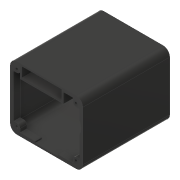
# Autodesk Inventor part: Case for Fan
Saved by Autodesk Inventor 2017 (Build 210142000, 142)
## iProperties
Created: 2016-08-11
Part Number: Case for Fan
Material: Generic
Document SubType Name: Modeling
Designer: ge937963
Density: 1 g/cm^3
Appearance: Smooth - Black
Mass: 36.4962 g
Surface Area: 460.668 cm^2
Volume: 36.4962 cm^3
Author: ge937963
Autodesk Inventor part; units mm, degrees
(part 1 of 2)
sketch "Sketch1" plane through (0, 0, 0) normal (0, 0, 1) x (1, 0, 0)
  line L0 (-32.8456, -23.6218) -> (-32.8456, 23.6218) projected
  arc A0 (-28.0831, 28.3843) -> (-32.8456, 23.6218) centre (-28.0831, 23.6218) ccw projected
  line L1 (-28.0831, 28.3843) -> (28.0831, 28.3843) projected
  arc A1 (32.8456, 23.6218) -> (28.0831, 28.3843) centre (28.0831, 23.6218) ccw projected
  line L2 (32.8456, 23.6218) -> (32.8456, -23.6218) projected
  arc A2 (28.0831, -28.3843) -> (32.8456, -23.6218) centre (28.0831, -23.6218) ccw projected
  line L3 (28.0831, -28.3843) -> (-28.0831, -28.3843) projected
  arc A3 (-32.8456, -23.6218) -> (-28.0831, -28.3843) centre (-28.0831, -23.6218) ccw projected
  arc A4 (-34.4331, -23.6218) -> (-28.0831, -29.9718) centre (-28.0831, -23.6218) ccw projected
  line L4 (-28.0831, -29.9718) -> (28.0831, -29.9718) projected
  arc A5 (28.0831, -29.9718) -> (34.4331, -23.6218) centre (28.0831, -23.6218) ccw projected
  line L5 (34.4331, -23.6218) -> (34.4331, 23.6218) projected
  arc A6 (34.4331, 23.6218) -> (28.0831, 29.9718) centre (28.0831, 23.6218) ccw projected
  line L6 (28.0831, 29.9718) -> (-28.0831, 29.9718) projected
  arc A7 (-28.0831, 29.9718) -> (-34.4331, 23.6218) centre (-28.0831, 23.6218) ccw projected
  line L7 (-34.4331, 23.6218) -> (-34.4331, -23.6218) projected
  point P0 (0, 0)
extrude "Extrusion1" add sketch "Sketch1" along normal blind 82.55
sketch "Sketch2" plane through (0, 0, 0) normal (0, 0, -1) x (-1, 0, 0)
  line L0 (32.8456, -23.6218) -> (32.8456, 23.6218) projected
  arc A0 (32.8456, 23.6218) -> (28.0831, 28.3843) centre (28.0831, 23.6218) ccw projected
  line L1 (28.0831, 28.3843) -> (-28.0831, 28.3843) projected
  arc A1 (-28.0831, 28.3843) -> (-32.8456, 23.6218) centre (-28.0831, 23.6218) ccw projected
  line L2 (-32.8456, 23.6218) -> (-32.8456, -23.6218) projected
  arc A2 (-32.8456, -23.6218) -> (-28.0831, -28.3843) centre (-28.0831, -23.6218) ccw projected
  line L3 (-28.0831, -28.3843) -> (28.0831, -28.3843) projected
  arc A3 (28.0831, -28.3843) -> (32.8456, -23.6218) centre (28.0831, -23.6218) ccw projected
  arc A4 (28.0831, -29.9718) -> (34.4331, -23.6218) centre (28.0831, -23.6218) ccw projected
  line L4 (28.0831, -29.9718) -> (-28.0831, -29.9718) projected
  arc A5 (-34.4331, -23.6218) -> (-28.0831, -29.9718) centre (-28.0831, -23.6218) ccw projected
  line L5 (-34.4331, -23.6218) -> (-34.4331, 23.6218) projected
  arc A6 (-28.0831, 29.9718) -> (-34.4331, 23.6218) centre (-28.0831, 23.6218) ccw projected
  line L6 (-28.0831, 29.9718) -> (28.0831, 29.9718) projected
  arc A7 (34.4331, 23.6218) -> (28.0831, 29.9718) centre (28.0831, 23.6218) ccw projected
  line L7 (34.4331, 23.6218) -> (34.4331, -23.6218) projected
  arc A8 (28.0831, -26.5428) -> (31.0041, -23.6218) centre (28.0831, -23.6218) ccw projected
  arc A9 (-31.0041, -23.6218) -> (-28.0831, -26.5428) centre (-28.0831, -23.6218) ccw projected
  arc A10 (-28.0831, 26.5428) -> (-31.0041, 23.6218) centre (-28.0831, 23.6218) ccw projected
  arc A11 (31.0041, 23.6218) -> (28.0831, 26.5428) centre (28.0831, 23.6218) ccw projected
  line L8 (32.4646, -23.6218) -> (32.4646, 23.6218)
  arc A12 (32.4646, 23.6218) -> (28.0831, 28.0033) centre (28.0831, 23.6218) ccw
  line L9 (28.0831, 28.0033) -> (-28.0831, 28.0033)
  arc A13 (-28.0831, 28.0033) -> (-32.4646, 23.6218) centre (-28.0831, 23.6218) ccw
  line L10 (-32.4646, 23.6218) -> (-32.4646, -23.6218)
  arc A14 (-32.4646, -23.6218) -> (-28.0831, -28.0033) centre (-28.0831, -23.6218) ccw
  line L11 (-28.0831, -28.0033) -> (28.0831, -28.0033)
  arc A15 (28.0831, -28.0033) -> (32.4646, -23.6218) centre (28.0831, -23.6218) ccw
  line L12 (28.0831, -26.5428) -> (-28.0831, -26.5428)
  line L13 (-31.0041, -23.6218) -> (-31.0041, 23.6218)
  line L14 (-28.0831, 26.5428) -> (28.0831, 26.5428)
  line L15 (31.0041, 23.6218) -> (31.0041, -23.6218)
  arc A16 (-31.3851, -23.6218) -> (-28.0831, -26.9238) centre (-28.0831, -23.6218) ccw
  line L16 (-31.3851, -23.6218) -> (-31.3851, 23.6218)
  arc A17 (-28.0831, 26.9238) -> (-31.3851, 23.6218) centre (-28.0831, 23.6218) ccw
  line L17 (-28.0831, 26.9238) -> (28.0831, 26.9238)
  arc A18 (31.3851, 23.6218) -> (28.0831, 26.9238) centre (28.0831, 23.6218) ccw
  line L18 (31.3851, 23.6218) -> (31.3851, -23.6218)
  arc A19 (28.0831, -26.9238) -> (31.3851, -23.6218) centre (28.0831, -23.6218) ccw
  line L19 (28.0831, -26.9238) -> (-28.0831, -26.9238)
  point P0 (0, 0)
  dimension "d2" = 0.381
  dimension "d3" = 0.381
  constraints: 24 end point, 16 point on circle, 8 centre point, 4 perpendicular, 2 tangent, 1 horizontal, 1 parallel, 14 other
  measures "d2" distance between parallel lines of L3 L11
  measures "d3" distance between parallel lines of L12 L19
extrude "Extrusion2" add sketch "Sketch2" along normal blind 3.175 contours A15 L11 A14 L10 A13 L9 A12 L8
sketch "Sketch3" plane through (0, 0, 0) normal (0, 0, 1) x (1, 0, 0)
  line L0 (31.3851, 23.6218) -> (31.3851, -23.6218) projected
  arc A0 (28.0831, -26.9238) -> (31.3851, -23.6218) centre (28.0831, -23.6218) ccw projected
  line L1 (28.0831, -26.9238) -> (-28.0831, -26.9238) projected
  arc A1 (-31.3851, -23.6218) -> (-28.0831, -26.9238) centre (-28.0831, -23.6218) ccw projected
  line L2 (-31.3851, -23.6218) -> (-31.3851, 23.6218) projected
  arc A2 (-28.0831, 26.9238) -> (-31.3851, 23.6218) centre (-28.0831, 23.6218) ccw projected
  line L3 (-28.0831, 26.9238) -> (28.0831, 26.9238) projected
  arc A3 (31.3851, 23.6218) -> (28.0831, 26.9238) centre (28.0831, 23.6218) ccw projected
  line L4 (-32.4646, -23.6218) -> (-32.4646, 23.6218) projected
  arc A4 (-32.4646, -23.6218) -> (-28.0831, -28.0033) centre (-28.0831, -23.6218) ccw projected
  line L5 (28.0831, -28.0033) -> (-28.0831, -28.0033) projected
  arc A5 (28.0831, -28.0033) -> (32.4646, -23.6218) centre (28.0831, -23.6218) ccw projected
  line L6 (32.4646, 23.6218) -> (32.4646, -23.6218) projected
  arc A6 (32.4646, 23.6218) -> (28.0831, 28.0033) centre (28.0831, 23.6218) ccw projected
  line L7 (-28.0831, 28.0033) -> (28.0831, 28.0033) projected
  arc A7 (-28.0831, 28.0033) -> (-32.4646, 23.6218) centre (-28.0831, 23.6218) ccw projected
  arc A8 (-28.0831, 28.3843) -> (-32.8456, 23.6218) centre (-28.0831, 23.6218) ccw projected
  line L8 (-28.0831, 28.3843) -> (28.0831, 28.3843) projected
  arc A9 (32.8456, 23.6218) -> (28.0831, 28.3843) centre (28.0831, 23.6218) ccw projected
  line L9 (32.8456, 23.6218) -> (32.8456, -23.6218) projected
  arc A10 (28.0831, -28.3843) -> (32.8456, -23.6218) centre (28.0831, -23.6218) ccw projected
  line L10 (28.0831, -28.3843) -> (-28.0831, -28.3843) projected
  arc A11 (-32.8456, -23.6218) -> (-28.0831, -28.3843) centre (-28.0831, -23.6218) ccw projected
  line L11 (-32.8456, -23.6218) -> (-32.8456, 23.6218) projected
  arc A12 (-34.4331, -23.6218) -> (-28.0831, -29.9718) centre (-28.0831, -23.6218) ccw projected
  line L12 (-28.0831, -29.9718) -> (28.0831, -29.9718) projected
  arc A13 (28.0831, -29.9718) -> (34.4331, -23.6218) centre (28.0831, -23.6218) ccw projected
  line L13 (34.4331, -23.6218) -> (34.4331, 23.6218) projected
  arc A14 (34.4331, 23.6218) -> (28.0831, 29.9718) centre (28.0831, 23.6218) ccw projected
  line L14 (28.0831, 29.9718) -> (-28.0831, 29.9718) projected
  arc A15 (-28.0831, 29.9718) -> (-34.4331, 23.6218) centre (-28.0831, 23.6218) ccw projected
  line L15 (-34.4331, 23.6218) -> (-34.4331, -23.6218) projected
  circle A16 centre (28.0831, 23.6218) radius 1.27 projected
  circle A17 centre (28.0831, 23.6218) radius 2.921 projected
  circle A18 centre (-28.0831, 23.6218) radius 1.27 projected
  circle A19 centre (-28.0831, 23.6218) radius 2.921 projected
  circle A20 centre (-28.0831, -23.6218) radius 1.27 projected
  circle A21 centre (-28.0831, -23.6218) radius 2.921 projected
  circle A22 centre (28.0831, -23.6218) radius 1.27 projected
  circle A23 centre (28.0831, -23.6218) radius 2.921 projected
  line L16 (28.0831, -26.9238) -> (-28.0831, -26.9238) projected
  line L17 (-28.0831, -26.9238) -> (-26.7209, -26.2058)
  line L18 (-31.3851, -23.6218) -> (-30.667, -22.2597)
  line L19 (28.0831, -26.9238) -> (26.7209, -26.2058)
  arc A24 (28.0831, -26.9238) -> (31.3851, -23.6218) centre (28.0831, -23.6218) ccw projected
  line L20 (31.3851, -23.6218) -> (30.667, -22.2597)
  line L21 (-28.0831, 26.9238) -> (28.0831, 26.9238) projected
  line L22 (28.0831, 26.9238) -> (26.7209, 26.2058)
  arc A25 (31.3851, 23.6218) -> (28.0831, 26.9238) centre (28.0831, 23.6218) ccw projected
  line L23 (31.3851, 23.6218) -> (31.3851, -23.6218) projected
  line L24 (31.3851, 23.6218) -> (30.667, 22.2597)
  arc A26 (-28.0831, 26.9238) -> (-31.3851, 23.6218) centre (-28.0831, 23.6218) ccw projected
  line L25 (-28.0831, 26.9238) -> (-26.7209, 26.2058)
  line L26 (-31.3851, -23.6218) -> (-31.3851, 23.6218) projected
  line L27 (-31.3851, 23.6218) -> (-30.667, 22.2597)
  circle A27 centre (-28.0831, 23.6218) radius 1.5875
  circle A28 centre (28.0831, 23.6218) radius 1.5875
  circle A29 centre (28.0831, -23.6218) radius 1.5875
  circle A30 centre (-28.0831, -23.6218) radius 1.5875
  point P0 (0, 0)
  dimension "d6" = 3.175
  dimension "d7" = 3.175
  dimension "d8" = 3.175
  dimension "d9" = 3.175
  constraints: 16 end point, 8 point on circle, 8 tangent, 4 centre point, 4 coincident
  measures "d6" diameter of A27
  measures "d7" diameter of A28
  measures "d8" diameter of A29
  measures "d9" diameter of A30
extrude "Extrusion3" add sketch "Sketch3" along normal blind 3.175 contours L24 A17 L22 A3 | A0 L19 A23 L20 | A17 | A23 | L25 A19 L27 A2 | A1 L18 A21 L17 | A19 | A21 | L4 A7 L7 A6 L6 A5 L5 A4 | L8 A9 L9 A10 L10 A11 L11 A8
chamfer "Chamfer1" distance 1.4478 angle 45 8 edges at (31.4507, 26.9894, 3.175) (32.8456, 0, 3.175) (31.4507, -26.9894, 3.175) (0, -28.3843, 3.175) (-31.4507, -26.9894, 3.175) (-32.8456, 0, 3.175) (-31.4507, 26.9894, 3.175) (0, 28.3843, 3.175)
sketch "Sketch4" plane through (32.8456, -23.6218, 82.55) normal (-1, 0, 0) x (0, 0, 1)
  line L0 (-74.51, 21.9075) -> (-74.51, -3.4925) projected
  point P0 (-82.55, 23.6218)
ref_plane "Work Plane1" through (-14.8768, -28.3843, 11.1882) normal (0, 0, 1) x (1, 0, 0)
sketch "Sketch5" plane through (-14.8768, -28.3843, 11.1882) normal (0, 0, 1) x (1, 0, 0)
  circle A0 centre (15.875, 6.985) radius 2.286 projected
  circle A1 centre (15.875, 20.955) radius 2.286 projected
  circle A2 centre (15.875, 13.97) radius 2.54 projected
  circle A3 centre (28.575, 3.175) radius 1.397 projected
  circle A4 centre (3.175, 3.175) radius 1.397 projected
  arc A5 (28.575, 13.97) -> (3.175, 13.97) centre (15.875, 13.97) ccw projected
  line L0 (28.575, 13.97) -> (28.575, 12.7) projected
  line L1 (28.575, 12.7) -> (31.3246, 7.9375) projected
  arc A6 (31.75, 6.35) -> (31.3246, 7.9375) centre (28.575, 6.35) ccw projected
  line L2 (31.75, 6.35) -> (31.75, 0) projected
  line L3 (31.75, 0) -> (0, 0) projected
  line L4 (0, 0) -> (0, 6.35) projected
  arc A7 (0.4254, 7.9375) -> (0, 6.35) centre (3.175, 6.35) ccw projected
  line L5 (0.4254, 7.9375) -> (3.175, 12.7) projected
  line L6 (3.175, 13.97) -> (3.175, 12.7) projected
  arc A8 (8.2603, 26.0592) -> (11.6942, 0.3079) centre (15.875, 13.97) ccw projected
  line L7 (0, 0) -> (6.35, 0)
  circle A9 centre (3.175, 3.175) radius 1.27
  circle A10 centre (28.575, 3.175) radius 1.27
  line L8 (0, 0) -> (0, 6.35)
  line L9 (6.35, 0) -> (31.75, 0)
  line L10 (0, 6.35) -> (31.75, 6.35)
  line L11 (31.75, 6.35) -> (31.75, 0)
  point P0 (14.8768, 28.3843)
  dimension "d15" = 6.35
  dimension "d16" = 2.54
  dimension "d17" = 2.54
  constraints: 10 end point, 2 centre point, 2 coincident, 2 perpendicular, 1 collinear, 1 point on line
  measures "d15" distance of L3.end L7.end
  measures "d16" diameter of A9
  measures "d17" diameter of A10
extrude "Extrusion4" add sketch "Sketch5" against normal blind 6.35 contours L10 A0 | A0 L10 L2 L3 L4 picked at (16.2273, 5.7626)
chamfer "Chamfer2" distance 1.905 angle 45 4 edges at (16.8732, -28.3843, 8.0132) (-14.8768, -28.3843, 8.0132) (-14.8768, -22.0343, 8.0132) (16.8732, -22.0343, 8.0132)
sketch "Sketch6" plane through (-14.8768, -28.3843, 4.8382) normal (0, 0, -1) x (-1, 0, 0)
  line L0 (-29.845, 6.35) -> (-1.905, 6.35) construction
  line L1 (-42.9599, 0) -> (13.2062, 0) projected
  line L2 (-24.765, 6.35) -> (-22.225, 6.35)
  line L3 (-22.225, 6.35) -> (-22.225, 0)
  line L4 (-22.225, 0) -> (-24.765, 0)
  line L5 (-24.765, 0) -> (-24.765, 6.35)
  line L6 (-9.525, 6.35) -> (-6.985, 6.35)
  line L7 (-6.985, 6.35) -> (-6.985, 0)
  line L8 (-6.985, 0) -> (-9.525, 0)
  line L9 (-9.525, 0) -> (-9.525, 6.35)
  line L10 (0, 1.905) -> (0, 4.445) projected
  line L11 (-31.75, 4.445) -> (-31.75, 1.905) projected
  point P0 (-14.8768, 28.3843)
  dimension "d24" = 2.54
  dimension "d25" = 12.7
  dimension "d26" = 2.54
  dimension "d27" = 2.54
  dimension "d28" = 6.985
  dimension "d29" = 6.985
  constraints: 16 end point, 4 parallel, 4 point on line, 2 horizontal, 2 perpendicular
  measures "d24" distance of L3.end L4.end
  measures "d25" distance between parallel lines of L9 L3
  measures "d26" distance between parallel lines of L9 L7
  measures "d27" distance between parallel lines of L3 L5
  measures "d28" distance between parallel lines of L10 L7
  measures "d29" distance between parallel lines of L11 L5
extrude "Extrusion5" add sketch "Sketch6" along normal blind 4.445
sketch "Sketch8" plane through (-7.8918, -28.3843, 4.8382) normal (-1, 0, 0) x (0, 0, 1)
  line L0 (-1.6632, 1.4605) -> (-4.445, 1.4605) projected
  line L1 (-1.6632, 1.4478) -> (-1.6632, 1.4605) projected
  line L2 (-0.2154, 0) -> (-1.6632, 1.4478) projected
  line L3 (0, 0) -> (-0.2154, 0) projected
  line L4 (0, 6.35) -> (0, 0) projected
  line L5 (0, 6.35) -> (-4.445, 6.35) projected
  line L6 (-4.445, 1.4605) -> (-4.445, 6.35) projected
  line L7 (-1.6632, 1.4605) -> (-4.445, 1.4605) projected
  line L8 (0, 6.35) -> (-4.445, 1.4605)
  point P0 (-4.8382, 28.3843)
  constraints: 2 end point
extrude "Extrusion6" cut sketch "Sketch8" against normal blind 25.4 contours L6 L5 L8
sketch "Sketch9" plane through (0, 0, 82.55) normal (0, 0, 1) x (1, 0, 0)
  line L0 (18.0306, 23.3043) -> (-18.0374, 23.3043) projected
  line L1 (18.0306, 23.3043) -> (18.0306, 27.1143) projected
  line L2 (-18.0374, 27.1143) -> (18.0306, 27.1143) projected
  line L3 (-18.0374, 23.3043) -> (-18.0374, 27.1143) projected
  line L4 (-18.0374, 22.0343) -> (18.0306, 22.0343) projected
  line L5 (-18.0374, 22.0343) -> (-18.0374, 18.2243) projected
  line L6 (18.0306, 18.2243) -> (-18.0374, 18.2243) projected
  line L7 (18.0306, 22.0343) -> (18.0306, 18.2243) projected
  line L8 (19.3006, 28.0033) -> (20.8881, 28.0033)
  line L9 (20.8881, 28.0033) -> (20.8881, 15.3668)
  line L10 (20.8881, 15.3668) -> (19.3006, 15.3668)
  line L11 (19.3006, 15.3668) -> (19.3006, 28.0033)
  line L12 (19.3006, 15.3668) -> (-20.8949, 15.3668)
  line L13 (-20.8949, 15.3668) -> (-20.8949, 16.9543)
  line L14 (-20.8949, 16.9543) -> (19.3006, 16.9543)
  line L15 (19.3006, 16.9543) -> (19.3006, 15.3668)
  line L16 (-28.0831, 28.0033) -> (28.0831, 28.0033) projected
  line L17 (-20.8949, 16.9543) -> (-19.3074, 16.9543)
  line L18 (-19.3074, 16.9543) -> (-19.3074, 28.0033)
  line L19 (-19.3074, 28.0033) -> (-20.8949, 28.0033)
  line L20 (-20.8949, 28.0033) -> (-20.8949, 16.9543)
  point P0 (0, 0)
  dimension "d34" = 1.5875
  dimension "d35" = 1.5875
  dimension "d36" = 1.5875
  dimension "d37" = 1.27
  dimension "d38" = 1.27
  dimension "d39" = 1.27
  constraints: 24 end point, 6 parallel, 3 horizontal, 3 perpendicular, 1 horizontal alignment, 1 point on line
  measures "d34" distance of L9.end L10.end
  measures "d35" distance of L14.end L10.end
  measures "d36" distance between parallel lines of L18 L20
  measures "d37" distance between parallel lines of L14 L6
  measures "d38" distance between parallel lines of L11 L7
  measures "d39" distance between parallel lines of L18 L5
extrude "Extrusion7" add sketch "Sketch9" against normal blind 63.5 contours L8 L9 L10 L11 | L11 L12 L13 L14 | L18 L14 L20 L16
fillet "Fillet1" radius 3.175 2 edges at (-20.8949, 15.3668, 50.8) (20.8881, 15.3668, 50.8)
sketch "Sketch10" plane through (19.3006, 28.0033, 82.55) normal (0, 1, 0) x (1, 0, 0)
  line L0 (-38.608, 0) -> (-40.1955, 0) projected
  line L1 (-38.608, 0) -> (-38.608, 63.5) projected
  line L2 (-40.1955, 63.5) -> (-38.608, 63.5) projected
  line L3 (-40.1955, 0) -> (-40.1955, 63.5) projected
  line L4 (1.5875, 0) -> (0, 0) projected
  line L5 (1.5875, 0) -> (1.5875, 63.5) projected
  line L6 (0, 63.5) -> (1.5875, 63.5) projected
  line L7 (0, 0) -> (0, 63.5) projected
  point P0 (-19.3006, 82.55)
extrude "Extrusion8" add sketch "Sketch10" along normal up to surface (1.9685 mm away)
fillet "Fillet2" radius 3.175 2 edges at (-20.8949, 28.3843, 50.8) (20.8881, 28.3843, 50.8)
fillet "Fillet3" radius 1.27 2 edges at (-19.3074, 16.9543, 50.8) (19.3006, 16.9543, 50.8)
sketch "Sketch11" plane through (0, 0, 19.05) normal (0, 0, -1) x (-1, 0, 0)
  arc A0 (-20.8881, 18.5418) -> (-17.7131, 15.3668) centre (-17.7131, 18.5418) ccw projected
  line L0 (-17.7131, 15.3668) -> (17.7199, 15.3668) projected
  arc A1 (17.7199, 15.3668) -> (20.8949, 18.5418) centre (17.7199, 18.5418) ccw projected
  line L1 (20.8949, 18.5418) -> (20.8949, 25.2093) projected
  arc A2 (24.0699, 28.3843) -> (20.8949, 25.2093) centre (24.0699, 25.2093) ccw projected
  line L2 (19.3074, 28.3843) -> (24.0699, 28.3843) projected
  line L3 (19.3074, 18.2243) -> (19.3074, 28.3843) projected
  arc A3 (18.0374, 16.9543) -> (19.3074, 18.2243) centre (18.0374, 18.2243) ccw projected
  line L4 (18.0374, 16.9543) -> (-18.0306, 16.9543) projected
  arc A4 (-19.3006, 18.2243) -> (-18.0306, 16.9543) centre (-18.0306, 18.2243) ccw projected
  line L5 (-19.3006, 18.2243) -> (-19.3006, 28.3843) projected
  line L6 (-24.0631, 28.3843) -> (-19.3006, 28.3843) projected
  arc A5 (-20.8881, 25.2093) -> (-24.0631, 28.3843) centre (-24.0631, 25.2093) ccw projected
  line L7 (-20.8881, 18.5418) -> (-20.8881, 25.2093) projected
  arc A6 (-20.8881, 25.2093) -> (-24.0631, 28.3843) centre (-24.0631, 25.2093) ccw projected
  line L8 (19.3074, 28.3843) -> (-24.0631, 28.3843)
  point P0 (0, 0)
  constraints: 2 end point, 1 horizontal, 1 tangent
extrude "Extrusion9" add sketch "Sketch11" along normal blind 1.5875
sketch "Sketch12" plane through (0, 0, 17.4625) normal (0, 0, -1) x (-1, 0, 0)
  line L0 (-19.3006, 18.2243) -> (-19.3006, 28.3843) projected
  line L1 (-19.3006, 19.4943) -> (-16.7606, 19.4943)
  line L2 (-16.7606, 19.4943) -> (-16.7606, 25.8443)
  line L3 (-16.7606, 25.8443) -> (-19.3006, 25.8443)
  line L4 (-19.3006, 25.8443) -> (-19.3006, 19.4943)
  point P0 (0, 0)
  dimension "d49" = 6.35
  dimension "d50" = 2.54
  dimension "d51" = 1.27
  constraints: 8 end point, 2 parallel, 1 horizontal, 1 perpendicular, 1 point on line
  measures "d49" distance of L1.end L2.end
  measures "d50" distance of L1.start L1.end
  measures "d51" distance from line of L0.start L1
extrude "Extrusion10" cut sketch "Sketch12" against normal blind 1.5875
fillet "Fillet4" radius 1.27 4 edges at (19.3006, 25.8443, 18.2563) (16.7606, 25.8443, 18.2563) (16.7606, 19.4943, 18.2563) (19.3006, 19.4943, 18.2563)
sketch "Sketch13" plane through (0, 0, 3.175) normal (0, 0, 1) x (1, 0, 0)
  line L0 (9.8882, -26.9238) -> (9.8882, -26.9365) projected
  line L1 (28.0831, -26.9365) -> (9.8882, -26.9365) projected
  arc A0 (28.0831, -26.9365) -> (31.3978, -23.6218) centre (28.0831, -23.6218) ccw projected
  line L2 (31.3978, 23.6218) -> (31.3978, -23.6218) projected
  arc A1 (31.3978, 23.6218) -> (28.0831, 26.9365) centre (28.0831, 23.6218) ccw construction
  line L3 (-28.0831, 26.9365) -> (28.0831, 26.9365) projected
  arc A2 (-28.0831, 26.9365) -> (-31.3978, 23.6218) centre (-28.0831, 23.6218) ccw construction
  line L4 (-31.3978, -23.6218) -> (-31.3978, 23.6218) projected
  arc A3 (-31.3978, -23.6218) -> (-28.0831, -26.9365) centre (-28.0831, -23.6218) ccw construction
  line L5 (-7.8918, -26.9365) -> (-28.0831, -26.9365) projected
  line L6 (-7.8918, -26.9365) -> (-7.8918, -26.9238) projected
  line L7 (-7.8918, -26.9238) -> (-28.0831, -26.9238) projected
  line L8 (-28.0831, -26.9238) -> (-26.7209, -26.2058) projected
  arc A4 (-26.7209, -26.2058) -> (-30.667, -22.2597) centre (-28.0831, -23.6218) ccw projected
  line L9 (-30.667, -22.2597) -> (-31.3851, -23.6218) projected
  line L10 (-31.3851, -23.6218) -> (-31.3851, 23.6218) projected
  line L11 (-31.3851, 23.6218) -> (-30.667, 22.2597) projected
  arc A5 (-30.667, 22.2597) -> (-26.7209, 26.2058) centre (-28.0831, 23.6218) ccw projected
  line L12 (-26.7209, 26.2058) -> (-28.0831, 26.9238) projected
  line L13 (-28.0831, 26.9238) -> (28.0831, 26.9238) projected
  line L14 (28.0831, 26.9238) -> (26.7209, 26.2058) projected
  arc A6 (26.7209, 26.2058) -> (30.667, 22.2597) centre (28.0831, 23.6218) ccw projected
  line L15 (30.667, 22.2597) -> (31.3851, 23.6218) projected
  line L16 (31.3851, 23.6218) -> (31.3851, -23.6218) projected
  line L17 (31.3851, -23.6218) -> (30.667, -22.2597) projected
  arc A7 (30.667, -22.2597) -> (26.7209, -26.2058) centre (28.0831, -23.6218) ccw projected
  line L18 (26.7209, -26.2058) -> (28.0831, -26.9238) projected
  line L19 (28.0831, -26.9238) -> (9.8882, -26.9238) projected
  circle A8 centre (-28.0831, 23.6218) radius 1.5875 construction
  circle A9 centre (-28.0831, -23.6218) radius 1.5875 construction
  circle A10 centre (28.0831, 23.6218) radius 1.5875 construction
  circle A11 centre (28.0831, -23.6218) radius 1.5875 construction
  arc A12 (30.667, -22.2597) -> (26.7209, -26.2058) centre (28.0831, -23.6218) ccw projected
  line L20 (28.0831, -20.7008) -> (31.3851, -20.7008)
  line L21 (25.1621, -23.6218) -> (25.1621, -26.9238)
  line L22 (28.0831, -26.9238) -> (9.8882, -26.9238) projected
  arc A13 (26.7209, 26.2058) -> (30.667, 22.2597) centre (28.0831, 23.6218) ccw projected
  line L23 (28.0831, 20.7008) -> (31.3851, 20.7008)
  line L24 (-28.0831, 26.9365) -> (28.0831, 26.9365) projected
  arc A14 (-26.7209, -26.2058) -> (-30.667, -22.2597) centre (-28.0831, -23.6218) ccw projected
  line L25 (-31.3978, -23.6218) -> (-31.3978, 23.6218) projected
  line L26 (-7.8918, -26.9365) -> (-28.0831, -26.9365) projected
  arc A15 (-30.667, 22.2597) -> (-26.7209, 26.2058) centre (-28.0831, 23.6218) ccw projected
  line L27 (-31.0041, 23.6218) -> (-31.0041, 26.9238)
  line L28 (-28.0831, 20.7008) -> (-31.3851, 20.7008)
  arc A16 (-30.667, 22.2597) -> (-26.7209, 26.2058) centre (-28.0831, 23.6218) ccw projected
  line L29 (-28.0831, -26.9238) -> (-26.7209, -26.2058) projected
  line L30 (-28.0831, -26.9238) -> (-28.0831, -26.9238)
  arc A17 (-26.7209, -26.2058) -> (-30.667, -22.2597) centre (-28.0831, -23.6218) ccw projected
  line L31 (-28.0831, 26.9238) -> (28.0831, 26.9238) projected
  line L32 (9.8882, -26.9238) -> (9.8882, -26.9365) projected
  line L33 (28.0831, -26.9365) -> (9.8882, -26.9365) projected
  arc A18 (28.0831, -26.9365) -> (31.3978, -23.6218) centre (28.0831, -23.6218) ccw projected
  line L34 (31.3978, 23.6218) -> (31.3978, -23.6218) projected
  arc A19 (31.3978, 23.6218) -> (28.0831, 26.9365) centre (28.0831, 23.6218) ccw projected
  line L35 (-28.0831, 26.9365) -> (28.0831, 26.9365) projected
  arc A20 (-28.0831, 26.9365) -> (-31.3978, 23.6218) centre (-28.0831, 23.6218) ccw projected
  line L36 (-31.3978, -23.6218) -> (-31.3978, 23.6218) projected
  arc A21 (-31.3978, -23.6218) -> (-28.0831, -26.9365) centre (-28.0831, -23.6218) ccw projected
  line L37 (-7.8918, -26.9365) -> (-28.0831, -26.9365) projected
  line L38 (-7.8918, -26.9365) -> (-7.8918, -26.9238) projected
  line L39 (-7.8918, -26.9238) -> (-28.0831, -26.9238) projected
  line L40 (-28.0831, -26.9238) -> (-26.7209, -26.2058) projected
  arc A22 (-26.7209, -26.2058) -> (-30.667, -22.2597) centre (-28.0831, -23.6218) ccw projected
  line L41 (-30.667, -22.2597) -> (-31.3851, -23.6218) projected
  line L42 (-31.3851, -23.6218) -> (-31.3851, 23.6218) projected
  line L43 (-31.3851, 23.6218) -> (-30.667, 22.2597) projected
  arc A23 (-30.667, 22.2597) -> (-26.7209, 26.2058) centre (-28.0831, 23.6218) ccw projected
  line L44 (-26.7209, 26.2058) -> (-28.0831, 26.9238) projected
  line L45 (-28.0831, 26.9238) -> (28.0831, 26.9238) projected
  line L46 (28.0831, 26.9238) -> (26.7209, 26.2058) projected
  arc A24 (26.7209, 26.2058) -> (30.667, 22.2597) centre (28.0831, 23.6218) ccw projected
  line L47 (30.667, 22.2597) -> (31.3851, 23.6218) projected
  line L48 (31.3851, 23.6218) -> (31.3851, -23.6218) projected
  line L49 (31.3851, -23.6218) -> (30.667, -22.2597) projected
  arc A25 (30.667, -22.2597) -> (26.7209, -26.2058) centre (28.0831, -23.6218) ccw projected
  line L50 (26.7209, -26.2058) -> (28.0831, -26.9238) projected
  line L51 (28.0831, -26.9238) -> (9.8882, -26.9238) projected
  circle A26 centre (-28.0831, 23.6218) radius 1.5875 projected
  circle A27 centre (-28.0831, -23.6218) radius 1.5875 projected
  circle A28 centre (28.0831, 23.6218) radius 1.5875 projected
  circle A29 centre (28.0831, -23.6218) radius 1.5875 projected
  line L52 (-25.1621, -23.6218) -> (-25.1621, -26.9238)
  line L53 (-7.8918, -26.9238) -> (-28.0831, -26.9238) projected
  line L54 (-31.3851, -20.7008) -> (-28.0831, -20.7008)
  line L55 (25.1621, 26.9238) -> (25.1621, 23.6218)
  line L56 (-25.1621, 26.9238) -> (-25.1621, 23.6218)
  arc A30 (26.7209, 26.2058) -> (30.667, 22.2597) centre (28.0831, 23.6218) ccw projected
  point P0 (0, 0)
  constraints: 20 end point, 17 point on circle, 10 perpendicular, 10 point on line, 9 tangent
ref_plane "Work Plane2" through (25.1621, 20.7008, 0) normal (0, 0, 1) x (1, 0, 0)
extrude "Extrusion11" add sketch "Sketch13" against normal up to surface (3.175 mm away) contours L21 A7 L18 L19 | L20 L16 L17 A7 | L23 A6 L15 L16 | L55 L13 L14 A6 | L56 A5 L12 L13 | L28 L10 L11 A5 | L7 L8 A4 L52 | L54 A4 L9 L10
sketch "Sketch14" plane through (0, 0, 82.55) normal (0, 0, 1) x (1, 0, 0)
  line L0 (9.8882, -26.9238) -> (9.8882, -26.9365) projected
  line L1 (28.0831, -26.9365) -> (9.8882, -26.9365) projected
  arc A0 (28.0831, -26.9365) -> (31.3978, -23.6218) centre (28.0831, -23.6218) ccw projected
  line L2 (31.3978, 23.6218) -> (31.3978, -23.6218) projected
  arc A1 (31.3978, 23.6218) -> (28.0831, 26.9365) centre (28.0831, 23.6218) ccw projected
  line L3 (-28.0831, 26.9365) -> (28.0831, 26.9365) projected
  arc A2 (-28.0831, 26.9365) -> (-31.3978, 23.6218) centre (-28.0831, 23.6218) ccw projected
  line L4 (-31.3978, -23.6218) -> (-31.3978, 23.6218) projected
  arc A3 (-31.3978, -23.6218) -> (-28.0831, -26.9365) centre (-28.0831, -23.6218) ccw projected
  line L5 (-7.8918, -26.9365) -> (-28.0831, -26.9365) projected
  line L6 (-7.8918, -26.9365) -> (-7.8918, -26.9238) projected
  line L7 (-7.8918, -26.9238) -> (-25.1621, -26.9238) projected
  line L8 (-25.1621, -26.9238) -> (-25.1621, -23.6218) projected
  arc A4 (-25.1621, -23.6218) -> (-28.0831, -20.7008) centre (-28.0831, -23.6218) ccw projected
  line L9 (-28.0831, -20.7008) -> (-31.3851, -20.7008) projected
  line L10 (-31.3851, -20.7008) -> (-31.3851, 20.7008) projected
  line L11 (-31.3851, 20.7008) -> (-28.0831, 20.7008) projected
  arc A5 (-28.0831, 20.7008) -> (-25.1621, 23.6218) centre (-28.0831, 23.6218) ccw projected
  line L12 (-25.1621, 23.6218) -> (-25.1621, 26.9238) projected
  line L13 (-25.1621, 26.9238) -> (25.1621, 26.9238) projected
  line L14 (25.1621, 26.9238) -> (25.1621, 23.6218) projected
  arc A6 (25.1621, 23.6218) -> (28.0831, 20.7008) centre (28.0831, 23.6218) ccw projected
  line L15 (28.0831, 20.7008) -> (31.3851, 20.7008) projected
  line L16 (31.3851, 20.7008) -> (31.3851, -20.7008) projected
  line L17 (31.3851, -20.7008) -> (28.0831, -20.7008) projected
  arc A7 (28.0831, -20.7008) -> (25.1621, -23.6218) centre (28.0831, -23.6218) ccw projected
  line L18 (25.1621, -23.6218) -> (25.1621, -26.9238) projected
  line L19 (25.1621, -26.9238) -> (9.8882, -26.9238) projected
  circle A8 centre (-28.0831, 23.6218) radius 1.5875 projected
  circle A9 centre (-28.0831, -23.6218) radius 1.5875 projected
  circle A10 centre (28.0831, 23.6218) radius 1.5875 projected
  circle A11 centre (28.0831, -23.6218) radius 1.5875 projected
  point P0 (0, 0)
ref_plane "Work Plane3" through (0, 0, 76.2) normal (0, 0, 1) x (1, 0, 0)
sketch "Sketch15" plane through (0, 0, 76.2) normal (0, 0, 1) x (1, 0, 0)
  arc A0 (25.1621, 23.6218) -> (28.0831, 20.7008) centre (28.0831, 23.6218) ccw projected
  line L0 (28.0831, 20.7008) -> (31.3851, 20.7008) projected
  line L1 (31.3978, 23.6218) -> (31.3978, -23.6218) construction
  arc A1 (31.3978, 23.6218) -> (28.0831, 26.9365) centre (28.0831, 23.6218) ccw projected
  circle A2 centre (28.0831, 23.6218) radius 1.5875 projected
  line L2 (-28.0831, 26.9365) -> (28.0831, 26.9365) construction
  line L3 (25.1621, 26.9238) -> (25.1621, 23.6218) projected
  circle A3 centre (-28.0831, 23.6218) radius 1.5875 projected
  arc A4 (-28.0831, 26.9365) -> (-31.3978, 23.6218) centre (-28.0831, 23.6218) ccw projected
  arc A5 (-28.0831, 20.7008) -> (-25.1621, 23.6218) centre (-28.0831, 23.6218) ccw projected
  line L4 (-25.1621, 23.6218) -> (-25.1621, 26.9238) projected
  line L5 (-31.3851, 20.7008) -> (-28.0831, 20.7008) projected
  line L6 (-31.3978, -23.6218) -> (-31.3978, 23.6218) construction
  line L7 (25.1621, -23.6218) -> (25.1621, -26.9238) projected
  arc A6 (28.0831, -20.7008) -> (25.1621, -23.6218) centre (28.0831, -23.6218) ccw projected
  line L8 (31.3851, -20.7008) -> (28.0831, -20.7008) projected
  arc A7 (28.0831, -28.3843) -> (32.8456, -23.6218) centre (28.0831, -23.6218) ccw projected
  arc A8 (28.0831, -28.3843) -> (32.8456, -23.6218) centre (28.0831, -23.6218) ccw projected
  circle A9 centre (28.0831, -23.6218) radius 1.5875 projected
  line L9 (28.0831, -26.9365) -> (9.8882, -26.9365) construction
  arc A10 (28.0831, -26.9365) -> (31.3978, -23.6218) centre (28.0831, -23.6218) ccw projected
  arc A11 (-31.3978, -23.6218) -> (-28.0831, -26.9365) centre (-28.0831, -23.6218) ccw projected
  line L10 (-7.8918, -26.9365) -> (-28.0831, -26.9365) construction
  line L11 (-25.1621, -26.9238) -> (-25.1621, -23.6218) projected
  circle A12 centre (-28.0831, -23.6218) radius 1.5875 projected
  arc A13 (-25.1621, -23.6218) -> (-28.0831, -20.7008) centre (-28.0831, -23.6218) ccw projected
  line L12 (-28.0831, -20.7008) -> (-31.3851, -20.7008) projected
  line L13 (25.1621, -26.9238) -> (25.1621, -26.9238)
  line L14 (-19.3074, 28.3843) -> (19.3006, 28.3843) projected
  line L15 (19.3006, 28.3843) -> (19.3006, 18.2243) projected
  arc A14 (18.0306, 16.9543) -> (19.3006, 18.2243) centre (18.0306, 18.2243) ccw projected
  line L16 (18.0306, 16.9543) -> (-18.0374, 16.9543) projected
  arc A15 (-19.3074, 18.2243) -> (-18.0374, 16.9543) centre (-18.0374, 18.2243) ccw projected
  line L17 (-19.3074, 18.2243) -> (-19.3074, 28.3843) projected
  line L18 (28.0831, 29.9718) -> (-28.0831, 29.9718) projected
  arc A16 (-28.0831, 29.9718) -> (-34.4331, 23.6218) centre (-28.0831, 23.6218) ccw projected
  line L19 (-34.4331, 23.6218) -> (-34.4331, -23.6218) projected
  arc A17 (-34.4331, -23.6218) -> (-28.0831, -29.9718) centre (-28.0831, -23.6218) ccw projected
  line L20 (-28.0831, -29.9718) -> (28.0831, -29.9718) projected
  arc A18 (28.0831, -29.9718) -> (34.4331, -23.6218) centre (28.0831, -23.6218) ccw projected
  line L21 (34.4331, -23.6218) -> (34.4331, 23.6218) projected
  arc A19 (34.4331, 23.6218) -> (28.0831, 29.9718) centre (28.0831, 23.6218) ccw projected
  line L22 (-20.8949, 25.2093) -> (-20.8949, 18.5418) projected
  arc A20 (-20.8949, 18.5418) -> (-17.7199, 15.3668) centre (-17.7199, 18.5418) ccw projected
  line L23 (-17.7199, 15.3668) -> (17.7131, 15.3668) projected
  arc A21 (17.7131, 15.3668) -> (20.8881, 18.5418) centre (17.7131, 18.5418) ccw projected
  line L24 (20.8881, 18.5418) -> (20.8881, 25.2093) projected
  arc A22 (24.0631, 28.3843) -> (20.8881, 25.2093) centre (24.0631, 25.2093) ccw projected
  line L25 (24.0631, 28.3843) -> (28.0831, 28.3843) projected
  arc A23 (32.8456, 23.6218) -> (28.0831, 28.3843) centre (28.0831, 23.6218) ccw projected
  line L26 (32.8456, 23.6218) -> (32.8456, -23.6218) projected
  arc A24 (28.0831, -28.3843) -> (32.8456, -23.6218) centre (28.0831, -23.6218) ccw projected
  line L27 (28.0831, -28.3843) -> (-28.0831, -28.3843) construction
  arc A25 (-32.8456, -23.6218) -> (-28.0831, -28.3843) centre (-28.0831, -23.6218) ccw projected
  line L28 (-32.8456, -23.6218) -> (-32.8456, 23.6218) projected
  arc A26 (-28.0831, 28.3843) -> (-32.8456, 23.6218) centre (-28.0831, 23.6218) ccw projected
  line L29 (-28.0831, 28.3843) -> (-24.0699, 28.3843) projected
  arc A27 (-20.8949, 25.2093) -> (-24.0699, 28.3843) centre (-24.0699, 25.2093) ccw projected
  line L30 (-28.0831, -26.9365) -> (28.0831, -26.9365)
  arc A28 (28.0831, -26.9365) -> (31.3978, -23.6218) centre (28.0831, -23.6218) ccw
  line L31 (31.3978, -23.6218) -> (31.3978, 23.6218)
  arc A29 (31.3978, 23.6218) -> (28.0831, 26.9365) centre (28.0831, 23.6218) ccw
  line L32 (28.0831, 26.9365) -> (21.399, 26.9365)
  line L33 (-21.4058, 26.9365) -> (-28.0831, 26.9365)
  arc A30 (-28.0831, 26.9365) -> (-31.3978, 23.6218) centre (-28.0831, 23.6218) ccw
  line L34 (-31.3978, 23.6218) -> (-31.3978, -23.6218)
  arc A31 (-31.3978, -23.6218) -> (-28.0831, -26.9365) centre (-28.0831, -23.6218) ccw
  line L35 (31.3851, -20.7008) -> (31.3978, -20.7008)
  line L36 (31.3851, 20.7008) -> (31.3978, 20.7008)
  line L37 (25.1621, -25.2728) -> (-25.1621, -25.2728)
  line L38 (-29.7341, -20.7008) -> (-29.7341, 20.7008)
  line L39 (29.7341, -20.7008) -> (29.7341, 20.7008)
  line L40 (25.1621, 25.2728) -> (-25.1621, 25.2728) construction
  line L41 (25.1621, 25.2728) -> (20.8881, 25.2093)
  line L42 (-25.1621, 23.6218) -> (-25.1621, 26.9238) projected
  line L43 (-20.8949, 25.2093) -> (-25.1621, 25.2728)
  point P0 (0, 0)
  constraints: 28 end point, 10 point on circle, 8 midpoint, 4 centre point, 4 point on line, 1 parallel, 1 perpendicular, 7 other
extrude "Extrusion12" add sketch "Sketch15" along normal blind 6.35 contours L3 L41 A22 L32 A1 L31 L36 L0 A0 | L0 L36 L31 L35 L8 L39 | L8 L35 L31 A10 L30 A11 L34 A4 L33 A27 L43 L4 A5 L5 L38 L12 A13 L11 L37 L7 A6
sketch "Sketch17" plane through (0, 0, 76.2) normal (0, 0, 1) x (1, 0, 0)
  line L0 (28.0831, 29.9718) -> (-28.0831, 29.9718) projected
  line L1 (28.0831, 29.9718) -> (-28.0831, 29.9718) projected
  arc A0 (34.4331, 23.6218) -> (28.0831, 29.9718) centre (28.0831, 23.6218) ccw projected
  line L2 (34.4331, -23.6218) -> (34.4331, 23.6218) projected
  arc A1 (28.0831, -29.9718) -> (34.4331, -23.6218) centre (28.0831, -23.6218) ccw projected
  line L3 (-28.0831, -29.9718) -> (28.0831, -29.9718) projected
  arc A2 (-34.4331, -23.6218) -> (-28.0831, -29.9718) centre (-28.0831, -23.6218) ccw projected
  line L4 (-34.4331, 23.6218) -> (-34.4331, -23.6218) projected
  arc A3 (-28.0831, 29.9718) -> (-34.4331, 23.6218) centre (-28.0831, 23.6218) ccw projected
  line L5 (28.0831, 29.9718) -> (-28.0831, 29.9718) projected
  point P0 (0, 0)
extrude "Extrusion13" add sketch "Sketch17" against normal blind 1.5875
sketch "Sketch18" plane through (0, 0, 76.2) normal (0, 0, 1) x (1, 0, 0)
  arc A0 (17.7131, 15.3668) -> (20.8881, 18.5418) centre (17.7131, 18.5418) ccw projected
  line L0 (-17.7199, 15.3668) -> (17.7131, 15.3668) projected
  arc A1 (-20.8949, 18.5418) -> (-17.7199, 15.3668) centre (-17.7199, 18.5418) ccw projected
  line L1 (-20.8949, 25.2093) -> (-20.8949, 18.5418) projected
  line L2 (-25.1621, 25.2728) -> (-20.8949, 25.2093) projected
  line L3 (-25.1621, 23.6218) -> (-25.1621, 25.2728) projected
  arc A2 (-28.0831, 20.7008) -> (-25.1621, 23.6218) centre (-28.0831, 23.6218) ccw projected
  line L4 (-29.7341, 20.7008) -> (-28.0831, 20.7008) projected
  line L5 (-29.7341, -20.7008) -> (-29.7341, 20.7008) projected
  line L6 (-28.0831, -20.7008) -> (-29.7341, -20.7008) projected
  arc A3 (-25.1621, -23.6218) -> (-28.0831, -20.7008) centre (-28.0831, -23.6218) ccw projected
  line L7 (-25.1621, -25.2728) -> (-25.1621, -23.6218) projected
  line L8 (25.1621, -25.2728) -> (-25.1621, -25.2728) projected
  line L9 (25.1621, -23.6218) -> (25.1621, -25.2728) projected
  arc A4 (28.0831, -20.7008) -> (25.1621, -23.6218) centre (28.0831, -23.6218) ccw projected
  line L10 (29.7341, -20.7008) -> (28.0831, -20.7008) projected
  line L11 (29.7341, 20.7008) -> (29.7341, -20.7008) projected
  line L12 (28.0831, 20.7008) -> (29.7341, 20.7008) projected
  arc A5 (25.1621, 23.6218) -> (28.0831, 20.7008) centre (28.0831, 23.6218) ccw projected
  line L13 (25.1621, 25.2728) -> (25.1621, 23.6218) projected
  line L14 (20.8881, 25.2093) -> (25.1621, 25.2728) projected
  line L15 (20.8881, 18.5418) -> (20.8881, 25.2093) projected
  line L16 (19.3006, 28.3843) -> (19.3006, 18.2243) projected
  line L17 (-19.3074, 28.3843) -> (19.3006, 28.3843) projected
  line L18 (-19.3074, 18.2243) -> (-19.3074, 28.3843) projected
  arc A6 (-19.3074, 18.2243) -> (-18.0374, 16.9543) centre (-18.0374, 18.2243) ccw projected
  line L19 (18.0306, 16.9543) -> (-18.0374, 16.9543) projected
  arc A7 (18.0306, 16.9543) -> (19.3006, 18.2243) centre (18.0306, 18.2243) ccw projected
  point P0 (0, 0)
extrude "Extrusion14" cut sketch "Sketch18" against normal blind 1.5875
sketch "Sketch20" plane through (0, 0, 82.55) normal (0, 0, 1) x (1, 0, 0)
  line L0 (-3.1826, -28.0764) -> (5.179, -28.0764) projected
  arc A0 (5.179, -28.0764) -> (8.6234, -2.3318) centre (0.9982, -14.4143) ccw projected
  line L1 (8.6234, -2.3318) -> (8.6234, 6.3272) projected
  line L2 (8.6234, 6.3272) -> (-6.6166, 6.3272) projected
  line L3 (-6.6166, 6.3272) -> (-6.6166, -2.3251) projected
  arc A1 (-6.6166, -2.3251) -> (-3.1826, -28.0764) centre (0.9982, -14.4143) ccw projected
  line L4 (-3.2284, -28.3843) -> (5.2248, -28.3843)
  arc A2 (5.2248, -28.3843) -> (8.9313, -2.1632) centre (0.9982, -14.4143) ccw
  line L5 (8.9313, -2.1632) -> (8.9313, 6.6351)
  line L6 (8.9313, 6.6351) -> (-6.9244, 6.6351)
  line L7 (-6.9244, 6.6351) -> (-6.9244, -2.1564)
  arc A3 (-6.9244, -2.1564) -> (-3.2284, -28.3843) centre (0.9982, -14.4143) ccw
  line L8 (-20.8949, 25.2093) -> (-20.8949, 18.5418) projected
  arc A4 (-20.8949, 18.5418) -> (-17.7199, 15.3668) centre (-17.7199, 18.5418) ccw projected
  line L9 (-17.7199, 15.3668) -> (17.7131, 15.3668) projected
  arc A5 (17.7131, 15.3668) -> (20.8881, 18.5418) centre (17.7131, 18.5418) ccw projected
  line L10 (20.8881, 18.5418) -> (20.8881, 25.2093) projected
  line L11 (20.8881, 25.2093) -> (25.1621, 25.2728) projected
  line L12 (25.1621, 25.2728) -> (25.1621, 23.6218) projected
  arc A6 (25.1621, 23.6218) -> (28.0831, 20.7008) centre (28.0831, 23.6218) ccw projected
  line L13 (28.0831, 20.7008) -> (29.7341, 20.7008) projected
  line L14 (29.7341, 20.7008) -> (29.7341, -20.7008) projected
  line L15 (29.7341, -20.7008) -> (28.0831, -20.7008) projected
  arc A7 (28.0831, -20.7008) -> (25.1621, -23.6218) centre (28.0831, -23.6218) ccw projected
  line L16 (25.1621, -23.6218) -> (25.1621, -25.2728) projected
  line L17 (25.1621, -25.2728) -> (-25.1621, -25.2728) projected
  line L18 (-25.1621, -25.2728) -> (-25.1621, -23.6218) projected
  arc A8 (-25.1621, -23.6218) -> (-28.0831, -20.7008) centre (-28.0831, -23.6218) ccw projected
  line L19 (-28.0831, -20.7008) -> (-29.7341, -20.7008) projected
  line L20 (-29.7341, -20.7008) -> (-29.7341, 20.7008) projected
  line L21 (-29.7341, 20.7008) -> (-28.0831, 20.7008) projected
  arc A9 (-28.0831, 20.7008) -> (-25.1621, 23.6218) centre (-28.0831, 23.6218) ccw projected
  line L22 (-25.1621, 23.6218) -> (-25.1621, 25.2728) projected
  line L23 (-25.1621, 25.2728) -> (-20.8949, 25.2093) projected
  circle A10 centre (28.0831, 23.6218) radius 1.5875 projected
  circle A11 centre (-28.0831, 23.6218) radius 1.5875 projected
  circle A12 centre (28.0831, -23.6218) radius 1.5875 projected
  circle A13 centre (-28.0831, -23.6218) radius 1.5875 projected
  line L24 (-19.3074, 28.3843) -> (19.3006, 28.3843) projected
  line L25 (19.3006, 28.3843) -> (19.3006, 18.2243) projected
  arc A14 (18.0306, 16.9543) -> (19.3006, 18.2243) centre (18.0306, 18.2243) ccw projected
  line L26 (18.0306, 16.9543) -> (-18.0374, 16.9543) projected
  arc A15 (-19.3074, 18.2243) -> (-18.0374, 16.9543) centre (-18.0374, 18.2243) ccw projected
  line L27 (-19.3074, 18.2243) -> (-19.3074, 28.3843) projected
  line L28 (28.0831, 29.9718) -> (-28.0831, 29.9718) projected
  arc A16 (-28.0831, 29.9718) -> (-34.4331, 23.6218) centre (-28.0831, 23.6218) ccw projected
  line L29 (-34.4331, 23.6218) -> (-34.4331, -23.6218) projected
  arc A17 (-34.4331, -23.6218) -> (-28.0831, -29.9718) centre (-28.0831, -23.6218) ccw projected
  line L30 (-28.0831, -29.9718) -> (28.0831, -29.9718) projected
  arc A18 (28.0831, -29.9718) -> (34.4331, -23.6218) centre (28.0831, -23.6218) ccw projected
  line L31 (34.4331, -23.6218) -> (34.4331, 23.6218) projected
  arc A19 (34.4331, 23.6218) -> (28.0831, 29.9718) centre (28.0831, 23.6218) ccw projected
  line L32 (-21.4058, 26.9365) -> (-28.0831, 26.9365) projected
  arc A20 (-28.0831, 26.9365) -> (-31.3978, 23.6218) centre (-28.0831, 23.6218) ccw projected
  line L33 (-31.3978, 23.6218) -> (-31.3978, -23.6218) projected
  arc A21 (-31.3978, -23.6218) -> (-28.0831, -26.9365) centre (-28.0831, -23.6218) ccw projected
  line L34 (-28.0831, -26.9365) -> (28.0831, -26.9365) projected
  arc A22 (28.0831, -26.9365) -> (31.3978, -23.6218) centre (28.0831, -23.6218) ccw projected
  line L35 (31.3978, -23.6218) -> (31.3978, 23.6218) projected
  arc A23 (31.3978, 23.6218) -> (28.0831, 26.9365) centre (28.0831, 23.6218) ccw projected
  line L36 (28.0831, 26.9365) -> (21.399, 26.9365) projected
  arc A24 (24.0631, 28.3843) -> (21.399, 26.9365) centre (24.0631, 25.2093) ccw projected
  line L37 (24.0631, 28.3843) -> (28.0831, 28.3843) projected
  arc A25 (32.8456, 23.6218) -> (28.0831, 28.3843) centre (28.0831, 23.6218) ccw projected
  line L38 (32.8456, 23.6218) -> (32.8456, -23.6218) projected
  arc A26 (28.0831, -28.3843) -> (32.8456, -23.6218) centre (28.0831, -23.6218) ccw projected
  line L39 (28.0831, -28.3843) -> (-28.0831, -28.3843) projected
  arc A27 (-32.8456, -23.6218) -> (-28.0831, -28.3843) centre (-28.0831, -23.6218) ccw projected
  line L40 (-32.8456, -23.6218) -> (-32.8456, 23.6218) projected
  arc A28 (-28.0831, 28.3843) -> (-32.8456, 23.6218) centre (-28.0831, 23.6218) ccw projected
  line L41 (-28.0831, 28.3843) -> (-24.0699, 28.3843) projected
  arc A29 (-21.4058, 26.9365) -> (-24.0699, 28.3843) centre (-24.0699, 25.2093) ccw projected
  line L42 (28.0831, -28.3843) -> (-28.0831, -28.3843) projected
  point P0 (0, 0)
  constraints: 8 end point, 4 point on circle, 2 centre point, 1 collinear, 5 other
extrude "Extrusion16" cut sketch "Sketch20" against normal blind 12.7 contours A1 L34 A0 L0 | L0 A0 L34 A2 L4 A3 A1 | L34 A3 L17 A1 | A1 L17 A0 L34 | A0 L17 A2 L34 | L17 A3 L7 L6 L5 A2 A0 L1 L2 L3 A1 | A1 L3 L2 L1 A0 L17
sketch "Sketch21" plane through (0, 0, -3.175) normal (0, 0, -1) x (-1, 0, 0)
  line L0 (-31.3851, -23.6218) -> (-31.3851, 23.6218) projected
  arc A0 (-28.0831, 26.9238) -> (-31.3851, 23.6218) centre (-28.0831, 23.6218) ccw projected
  line L1 (-28.0831, 26.9238) -> (28.0831, 26.9238) projected
  arc A1 (31.3851, 23.6218) -> (28.0831, 26.9238) centre (28.0831, 23.6218) ccw projected
  line L2 (31.3851, 23.6218) -> (31.3851, -23.6218) projected
  arc A2 (28.0831, -26.9238) -> (31.3851, -23.6218) centre (28.0831, -23.6218) ccw projected
  line L3 (28.0831, -26.9238) -> (-28.0831, -26.9238) projected
  arc A3 (-31.3851, -23.6218) -> (-28.0831, -26.9238) centre (-28.0831, -23.6218) ccw projected
  line L4 (32.4646, -23.6218) -> (32.4646, 23.6218) projected
  arc A4 (32.4646, 23.6218) -> (28.0831, 28.0033) centre (28.0831, 23.6218) ccw projected
  line L5 (28.0831, 28.0033) -> (-28.0831, 28.0033) projected
  arc A5 (-28.0831, 28.0033) -> (-32.4646, 23.6218) centre (-28.0831, 23.6218) ccw projected
  line L6 (-32.4646, 23.6218) -> (-32.4646, -23.6218) projected
  arc A6 (-32.4646, -23.6218) -> (-28.0831, -28.0033) centre (-28.0831, -23.6218) ccw projected
  line L7 (-28.0831, -28.0033) -> (28.0831, -28.0033) projected
  arc A7 (28.0831, -28.0033) -> (32.4646, -23.6218) centre (28.0831, -23.6218) ccw projected
  line L8 (-28.0831, 27.7493) -> (28.0831, 27.7493)
  arc A8 (32.2106, 23.6218) -> (28.0831, 27.7493) centre (28.0831, 23.6218) ccw
  line L9 (32.2106, 23.6218) -> (32.2106, -23.6218)
  arc A9 (28.0831, -27.7493) -> (32.2106, -23.6218) centre (28.0831, -23.6218) ccw
  line L10 (28.0831, -27.7493) -> (-28.0831, -27.7493)
  arc A10 (-32.2106, -23.6218) -> (-28.0831, -27.7493) centre (-28.0831, -23.6218) ccw
  line L11 (-32.2106, -23.6218) -> (-32.2106, 23.6218)
  arc A11 (-28.0831, 27.7493) -> (-32.2106, 23.6218) centre (-28.0831, 23.6218) ccw
  line L12 (28.0831, 27.1778) -> (-28.0831, 27.1778)
  arc A12 (-28.0831, 27.1778) -> (-31.6391, 23.6218) centre (-28.0831, 23.6218) ccw
  line L13 (-31.6391, 23.6218) -> (-31.6391, -23.6218)
  arc A13 (-31.6391, -23.6218) -> (-28.0831, -27.1778) centre (-28.0831, -23.6218) ccw
  line L14 (-28.0831, -27.1778) -> (28.0831, -27.1778)
  arc A14 (28.0831, -27.1778) -> (31.6391, -23.6218) centre (28.0831, -23.6218) ccw
  line L15 (31.6391, -23.6218) -> (31.6391, 23.6218)
  arc A15 (31.6391, 23.6218) -> (28.0831, 27.1778) centre (28.0831, 23.6218) ccw
  line L16 (-28.0831, 28.3843) -> (28.0831, 28.3843) projected
  point P0 (0, 0)
  dimension "d69" = 0.254
  dimension "d70" = 0.254
  constraints: 16 end point, 16 point on circle, 8 centre point, 14 other
  measures "d69" distance between parallel lines of L8 L5
  measures "d70" distance between parallel lines of L1 L12
extrude "Extrusion17" cut sketch "Sketch21" against normal up to surface (3.175 mm away)
sketch "Sketch22" plane through (34.4331, -23.6218, 0) normal (1, 0, 0) x (0, 0, -1)
  line L0 (38.6107, 68.6676) -> (0, 68.6676)
  line L1 (0, 68.6676) -> (0, -22.5168)
  line L2 (0, -22.5168) -> (38.6107, -22.5168)
  line L3 (38.6107, -22.5168) -> (38.6107, 68.6676)
  line L4 (0, 0) -> (0, 47.2436) projected
  point P0 (0, 23.6218)
  point P1 (0, 23.6218)
  constraints: 8 end point, 2 parallel, 1 horizontal, 1 midpoint, 1 perpendicular, 1 point on line
extrude "Extrusion18" cut sketch "Sketch22" against normal through all
sketch "Sketch23" plane through (0, 0, 82.55) normal (0, 0, 1) x (1, 0, 0)
  arc A0 (5.2248, -28.3843) -> (8.4961, -26.9365) centre (0.9982, -14.4143) ccw projected
  line L0 (28.0831, -28.3843) -> (5.2248, -28.3843) projected
  arc A1 (28.0831, -28.3843) -> (32.8456, -23.6218) centre (28.0831, -23.6218) ccw projected
  line L1 (32.8456, 23.6218) -> (32.8456, -23.6218) projected
  arc A2 (32.8456, 23.6218) -> (28.0831, 28.3843) centre (28.0831, 23.6218) ccw projected
  line L2 (24.0631, 28.3843) -> (28.0831, 28.3843) projected
  arc A3 (24.0631, 28.3843) -> (21.399, 26.9365) centre (24.0631, 25.2093) ccw projected
  line L3 (28.0831, 26.9365) -> (21.399, 26.9365) projected
  arc A4 (31.3978, 23.6218) -> (28.0831, 26.9365) centre (28.0831, 23.6218) ccw projected
  line L4 (31.3978, -23.6218) -> (31.3978, 23.6218) projected
  arc A5 (28.0831, -26.9365) -> (31.3978, -23.6218) centre (28.0831, -23.6218) ccw projected
  line L5 (8.4961, -26.9365) -> (28.0831, -26.9365) projected
  arc A6 (-6.4998, -26.9365) -> (-3.2284, -28.3843) centre (0.9982, -14.4143) ccw projected
  line L6 (-28.0831, -26.9365) -> (-6.4998, -26.9365) projected
  arc A7 (-31.3978, -23.6218) -> (-28.0831, -26.9365) centre (-28.0831, -23.6218) ccw projected
  line L7 (-31.3978, 23.6218) -> (-31.3978, -23.6218) projected
  arc A8 (-28.0831, 26.9365) -> (-31.3978, 23.6218) centre (-28.0831, 23.6218) ccw projected
  line L8 (-21.4058, 26.9365) -> (-28.0831, 26.9365) projected
  arc A9 (-21.4058, 26.9365) -> (-24.0699, 28.3843) centre (-24.0699, 25.2093) ccw projected
  line L9 (-28.0831, 28.3843) -> (-24.0699, 28.3843) projected
  arc A10 (-28.0831, 28.3843) -> (-32.8456, 23.6218) centre (-28.0831, 23.6218) ccw projected
  line L10 (-32.8456, -23.6218) -> (-32.8456, 23.6218) projected
  arc A11 (-32.8456, -23.6218) -> (-28.0831, -28.3843) centre (-28.0831, -23.6218) ccw projected
  line L11 (-3.2284, -28.3843) -> (-28.0831, -28.3843) projected
  arc A12 (-20.8949, 25.2093) -> (-24.0699, 28.3843) centre (-24.0699, 25.2093) ccw projected
  line L12 (-24.0699, 28.3843) -> (-20.8949, 28.3843)
  line L13 (-20.8949, 28.3843) -> (-20.8949, 16.3728)
  line L14 (-20.8949, 16.3728) -> (-12.0493, 5.1975)
  line L15 (-12.0493, 5.1975) -> (24.0631, 8.5981)
  line L16 (20.8881, 25.2093) -> (25.1621, 25.2728) projected
  line L17 (24.0631, 8.5981) -> (20.8881, 25.2093)
  line L18 (20.8881, 25.2093) -> (20.8881, 28.3843)
  line L19 (28.0831, 28.3843) -> (-28.0831, 28.3843) projected
  line L20 (24.0631, 28.3843) -> (20.8881, 28.3843)
  arc A13 (-8.7547, -25.2728) -> (-3.2284, -28.3843) centre (0.9982, -14.4143) ccw projected
  arc A14 (5.2248, -28.3843) -> (10.751, -25.2728) centre (0.9982, -14.4143) ccw projected
  line L21 (-3.2284, -28.3843) -> (5.2248, -28.3843)
  point P0 (0, 0)
  constraints: 16 end point, 2 horizontal, 2 perpendicular, 2 point on line, 1 parallel, 1 point on circle, 1 tangent
extrude "Extrusion19" cut sketch "Sketch23" against normal blind 25.4 contours L21 A6 L6 A7 L7 A8 L8 A12 L13 L14 L15 L17 L18 L19 A3 L3 A4 L4 A5 L5 A0 | A0 L5 A5 L4 A4 L3 A3 L2 A2 L1 A1 L0 | L11 A11 L10 A10 L9 A9 L8 A8 L7 A7 L6 A6 | L12 L13 A12 A9
sketch "Sketch24" plane through (0, 0, 82.55) normal (0, 0, 1) x (1, 0, 0)
  arc A0 (-34.4331, -23.6218) -> (-28.0831, -29.9718) centre (-28.0831, -23.6218) ccw projected
  line L0 (-34.4331, 23.6218) -> (-34.4331, -23.6218) projected
  arc A1 (-28.0831, 29.9718) -> (-34.4331, 23.6218) centre (-28.0831, 23.6218) ccw projected
  line L1 (28.0831, 29.9718) -> (-28.0831, 29.9718) projected
  arc A2 (34.4331, 23.6218) -> (28.0831, 29.9718) centre (28.0831, 23.6218) ccw projected
  line L2 (34.4331, -23.6218) -> (34.4331, 23.6218) projected
  arc A3 (28.0831, -29.9718) -> (34.4331, -23.6218) centre (28.0831, -23.6218) ccw projected
  line L3 (-28.0831, -29.9718) -> (28.0831, -29.9718) projected
  circle A4 centre (28.0831, -23.6218) radius 1.5875 projected
  circle A5 centre (28.0831, 23.6218) radius 1.5875 projected
  circle A6 centre (-28.0831, 23.6218) radius 1.5875 projected
  line L4 (25.1621, -26.9238) -> (-25.1621, -26.9238) projected
  line L5 (25.1621, -26.9238) -> (25.1621, -23.6218) projected
  arc A7 (28.0831, -20.7008) -> (25.1621, -23.6218) centre (28.0831, -23.6218) ccw projected
  line L6 (28.0831, -20.7008) -> (31.3851, -20.7008) projected
  line L7 (31.3851, 20.7008) -> (31.3851, -20.7008) projected
  line L8 (31.3851, 20.7008) -> (28.0831, 20.7008) projected
  arc A8 (25.1621, 23.6218) -> (28.0831, 20.7008) centre (28.0831, 23.6218) ccw projected
  line L9 (25.1621, 23.6218) -> (25.1621, 26.9238) projected
  line L10 (-25.1621, 26.9238) -> (25.1621, 26.9238) projected
  line L11 (-25.1621, 26.9238) -> (-25.1621, 23.6218) projected
  arc A9 (-28.0831, 20.7008) -> (-25.1621, 23.6218) centre (-28.0831, 23.6218) ccw projected
  line L12 (-28.0831, 20.7008) -> (-31.3851, 20.7008) projected
  line L13 (-31.3851, -20.7008) -> (-31.3851, 20.7008) projected
  line L14 (-31.3851, -20.7008) -> (-28.0831, -20.7008) projected
  arc A10 (-25.1621, -23.6218) -> (-28.0831, -20.7008) centre (-28.0831, -23.6218) ccw projected
  line L15 (-25.1621, -23.6218) -> (-25.1621, -26.9238) projected
  circle A11 centre (-28.0831, -23.6218) radius 1.5875 projected
  point P0 (0, 0)
sketch "Sketch25" plane through (0, 0, 82.55) normal (0, 0, 1) x (1, 0, 0)
  line L0 (28.0831, 28.3843) -> (-28.0831, 28.3843) projected
  line L1 (-24.7241, 8.3085) -> (24.7953, 8.3085)
  line L2 (24.7953, 8.3085) -> (24.7953, 28.3843)
  line L3 (24.7953, 28.3843) -> (-24.7241, 28.3843)
  line L4 (-24.7241, 28.3843) -> (-24.7241, 8.3085)
  point P0 (0, 0)
  constraints: 8 end point, 2 parallel, 1 horizontal, 1 perpendicular, 1 point on line
extrude "Extrusion20" cut sketch "Sketch25" against normal up to surface (77.9272 mm away)
extrude "Extrusion21" add sketch "Sketch24" against normal blind 6.35
sketch "Sketch26" plane through (0, 0, 82.55) normal (0, 0, 1) x (1, 0, 0)
  line L0 (-10.795, -13.6783) -> (10.795, -13.6783)
  line L1 (10.795, -13.6783) -> (10.795, -28.3843)
  line L2 (10.795, -28.3843) -> (-10.795, -28.3843)
  line L3 (-10.795, -28.3843) -> (-10.795, -13.6783)
  point P0 (0, 0)
  point P1 (0, -28.3843)
  point P2 (-16.7818, -28.3843)
  dimension "d81" = 21.59
  constraints: 8 end point, 2 parallel, 1 horizontal, 1 horizontal alignment, 1 midpoint, 1 perpendicular, 1 vertical alignment
  measures "d81" distance of L1.end L2.end
extrude "Extrusion22" cut sketch "Sketch26" against normal blind 6.35